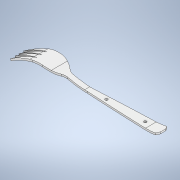
# Autodesk Inventor part: fork
Saved by Autodesk Inventor 2022 (Build 260153000, 153)
## iProperties
Created: 2022-10-22
Part Number: fork
Material: ポリスチレン
Document SubType Name: Modeling
Designer: Yazawa
Density: 1.021 g/cm^3
Appearance: 滑らか - 白
Mass: 5.29286 g
Surface Area: 61.1423 cm^2
Volume: 5.18399 cm^3
Author: Yazawa
Autodesk Inventor part; units mm, degrees
ref_plane "YZ Plane" through (0, 0, 0) normal (1, 0, 0) x (0, 1, 0)
ref_plane "XZ Plane" through (0, 0, 0) normal (0, 1, 0) x (-1, 0, 0)
ref_plane "XY Plane" through (0, 0, 0) normal (0, 0, 1) x (1, 0, 0)
sketch "スケッチ2" plane through (0, 0, 0) normal (0, 0, 1) x (1, 0, 0)
  arc A0 (-18.0723, 8.4646) -> (-44.4977, 8.2149) centre (-30.9427, -27.8877) ccw
  arc A1 (-18.0723, 8.4646) -> (17.6933, 1.1527) centre (26.0163, 132.9927) ccw
  arc A2 (99.6933, 1.1527) -> (115.4364, 3.2181) centre (99.6933, 62.1838) ccw
  arc A3 (-44.4977, 8.2149) -> (-72.801, -6.8342) centre (-0.878, -107.9623) ccw
  line L0 (17.6933, 1.1527) -> (99.6933, 1.1527)
  arc A4 (-43.7244, 6.1553) -> (-71.526, -8.627) centre (-0.878, -107.9623) ccw
  arc A5 (-18.8066, 6.3908) -> (-43.7244, 6.1553) centre (-30.9427, -27.8877) ccw
  arc A6 (-18.8066, 6.3908) -> (17.6242, -1.0473) centre (26.0163, 132.9927) ccw
  line L1 (17.6242, -1.0473) -> (99.6933, -1.0473)
  arc A7 (99.6933, -1.0473) -> (116.0039, 1.0926) centre (99.6933, 62.1838) ccw
  line L2 (-72.801, -6.8342) -> (-71.526, -8.627)
  line L3 (115.4364, 3.2181) -> (116.0039, 1.0926)
  point P0 (0, 0)
  dimension "d19" = 82
  dimension "d26" = 132.1025
  dimension "d27" = 38.5634
  dimension "d28" = 124.096
  dimension "d29" = 14.842
  dimension "d30" = 40.075
  dimension "d31" = 15.884
  dimension "d32" = 14.949
  dimension "d33" = 61.0311
  dimension "d34" = 2.2
  constraints: 16 point on circle, 8 centre point, 8 end point, 2 tangent, 1 horizontal, 4 other
  measures "d19" distance of L0.start L0.end
  measures "d26" radius of A1
  measures "d27" radius of A0
  measures "d28" radius of A3
  measures "d33" radius of A2
  measures "d34" radial gap between concentric circles of A0 A5
extrude "押し出し2" add sketch "スケッチ2" along normal blind 24.32
sketch "スケッチ3" plane through (17.6242, -1.0473, 0) normal (0, -1, 0) x (1, 0, 0)
  line L0 (98.3797, 0) -> (98.3797, 24.32) projected
  arc A0 (-45.5784, 24.32) -> (-58.4546, 24.1908) centre (-45.5784, -617.2518) ccw
  line L1 (-61.3487, 24.32) -> (-36.4308, 24.32) projected
  arc A1 (-27.6481, 17.7751) -> (-45.5784, 24.32) centre (-45.5784, -3.5132) ccw
  arc A2 (-27.6481, 17.7751) -> (-21.3876, 15.4513) centre (-21.2803, 25.3354) ccw
  arc A3 (95.2752, 19.5094) -> (3.1956, 15.4513) centre (209.2083, -3612.3091) ccw
  line L2 (97.8122, 0) -> (97.8122, 24.32) projected
  arc A4 (98.3797, 12.16) -> (95.2752, 19.5094) centre (88.128, 12.16) ccw
  line L3 (-21.3876, 15.4513) -> (3.1956, 15.4513)
  line L4 (-90.4253, 0) -> (-90.4253, 24.32) projected
  line L5 (-58.4546, 24.1908) -> (-90.4253, 20.6993)
  line L6 (-90.4253, 20.6993) -> (-58.4546, 18.5366)
  line L7 (-58.4546, 18.5366) -> (-90.4253, 14.6253)
  line L8 (-90.4253, 14.6253) -> (-58.4546, 12.16)
  line L9 (-58.4546, 12.16) -> (98.3797, 12.16)
  arc A5 (-58.4546, 0.1292) -> (-45.5784, 0) centre (-45.5784, 641.5718) ccw
  arc A6 (-45.5784, 0) -> (-27.6481, 6.5449) centre (-45.5784, 27.8332) ccw
  arc A7 (-21.3876, 8.8687) -> (-27.6481, 6.5449) centre (-21.2803, -1.0154) ccw
  arc A8 (3.1956, 8.8687) -> (95.2752, 4.8106) centre (209.2083, 3636.6291) ccw
  arc A9 (95.2752, 4.8106) -> (98.3797, 12.16) centre (88.128, 12.16) ccw
  line L10 (-21.3876, 8.8687) -> (3.1956, 8.8687)
  line L11 (-58.4546, 0.1292) -> (-90.4253, 3.6207)
  line L12 (-90.4253, 3.6207) -> (-58.4546, 5.7834)
  line L13 (-58.4546, 5.7834) -> (-90.4253, 9.6947)
  line L14 (-90.4253, 9.6947) -> (-58.4546, 12.16)
  point P0 (97.8122, 12.16)
  point P1 (97.8122, 8.7964)
  point P2 (97.8122, 15.5236)
  constraints: 22 end point, 22 point on circle, 14 symmetric about line, 10 centre point, 4 tangent, 3 vertical alignment, 2 horizontal, 2 midpoint, 2 point on line, 15 other
extrude "押し出し3" cut sketch "スケッチ3" along normal mid plane 24.32 contours A1 A2 L3 A3 A4 L2 L9 L8 L7 L6 L5 A0 | L14 L9 L2 A9 A8 L10 A7 A6 A5 L11 L12 L13 keep common part
sketch "スケッチ4" plane through (17.6242, -1.0473, 8.8687) normal (0, -1, 0) x (1, 0, 0)
  line L0 (97.8122, 6.6548) -> (97.8122, -0.0723) projected
  point P0 (-17.6242, -8.8687)
  point P1 (74.8122, 3.2913)
  point P2 (97.8122, 3.2913)
  point P3 (24.8122, 3.2913)
  dimension "d39" = 23
  dimension "d47" = 50
  constraints: 2 horizontal alignment, 1 midpoint
  measures "d39" distance of point (97.812, 3.291) point (74.812, 3.291)
  measures "d47" distance of point (74.812, 3.291) point (24.812, 3.291)
hole "穴1" at (92.4364, -1.0473, 12.16) at (42.4364, -1.0473, 12.16) direction (0, 1, 0) diameter 3.4 end through all clearance for "Countersunk Flat Head Screw ISO 2009/7046" size "M3" standard "ISO"
